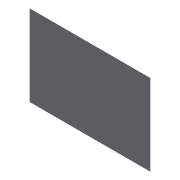
# Autodesk Inventor part: Side104x700
Saved by Autodesk Inventor 2014 SP1 (Build 180222100, 222)
## iProperties
Created: 2015-02-11
Part Number: Side104x700
Material: Generic
Document SubType Name: Modeling
Designer: Simen
Density: 1 g/cm^3
Appearance: Default
Author: Simen
Autodesk Inventor part; units mm, degrees
ref_plane "YZ Plane" through (0, 0, 0) normal (1, 0, 0) x (0, 1, 0)
ref_plane "XZ Plane" through (0, 0, 0) normal (0, 1, 0) x (-1, 0, 0)
ref_plane "XY Plane" through (0, 0, 0) normal (0, 0, 1) x (1, 0, 0)
sketch "Sketch1" plane through (0, 0, 0) normal (0, 1, 0) x (-1, 0, 0)
  line L0 (-89.6936, 55.1708) -> (950.3064, 55.1708)
  line L1 (950.3064, 55.1708) -> (950.3064, -644.8292)
  line L2 (950.3064, -644.8292) -> (-89.6936, -644.8292)
  line L3 (-89.6936, -644.8292) -> (-89.6936, 55.1708)
  point P0 (0, 0)
  dimension "d0" = 1040
  dimension "d1" = 700
  constraints: 8 end point, 2 parallel, 1 horizontal, 1 perpendicular
  measures "d0" distance of L1.end L2.end
  measures "d1" distance of L0.end L1.end
extrude "Extrusion1" add sketch "Sketch1" along normal blind 0.8
body "Solid1"
